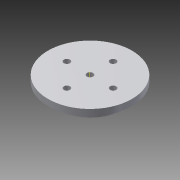
# Autodesk Inventor part: TapaPosterior
Saved by Autodesk Inventor 2013 (Build 170138000, 138)
## iProperties
Created: 2013-06-25
Part Number: TapaPosterior
Material: Genérico
Document SubType Name: Modeling
Designer: usuario
Density: 1 g/cm^3
Author: usuario
Autodesk Inventor part; units mm, degrees
ref_plane "YZ Plane" through (0, 0, 0) normal (1, 0, 0) x (0, 1, 0)
ref_plane "XY Plane" through (0, 0, 0) normal (0, 0, 1) x (1, 0, 0)
sketch "Boceto1" plane through (0, 0, 0) normal (0, 0, 1) x (1, 0, 0)
  circle A0 centre (0, 0) radius 13.5
  dimension "d0" = 27
  constraints: 1 centre point, 1 coincident
  measures "d0" diameter of A0
extrude "Extrusión1" add sketch "Boceto1" along normal blind 2
sketch "Boceto2" plane through (0, 0, 0) normal (0, 0, -1) x (-1, 0, 0)
  circle A0 centre (0, 0) radius 13.5 projected
  circle A1 centre (0, 0) radius 11.23
  dimension "d3" = 22.46
  constraints: 1 centre point, 1 coincident
  measures "d3" diameter of A1
extrude "Extrusión2" add sketch "Boceto2" along normal blind 2 contours A1
sketch "Boceto3" plane through (0, 0, -2) normal (0, 0, -1) x (-1, 0, 0)
  circle A0 centre (0, 0) radius 11.23 projected
  circle A1 centre (0, 0) radius 5.92
  dimension "d6" = 11.84
  constraints: 1 centre point, 1 coincident
  measures "d6" diameter of A1
extrude "Extrusión3" add sketch "Boceto3" along normal blind 2 contours A1
sketch "Boceto4" plane through (0, 0, -4) normal (0, 0, -1) x (-1, 0, 0)
  circle A0 centre (0, 0) radius 5.92 projected
  circle A1 centre (0, 0) radius 3.925
  dimension "d9" = 7.85
  constraints: 1 centre point, 1 coincident
  measures "d9" diameter of A1
extrude "Extrusión4" add sketch "Boceto4" along normal blind 2.5 contours A1
hole "Hole1" at (0, 0, 2) direction (0, 0, -1) diameter 2.02 end through all
hole "Hole2" at (0, 0, -6.5) direction (0, 0, 1) diameter 5.2 depth 2.5
ref_plane "Plano de trabajo1" through (0, 3.925, -4) normal (0, 1, 0) x (-1, 0, 0)
sketch "Boceto11" plane through (0, 3.925, -4) normal (0, 1, 0) x (-1, 0, 0)
  line L0 (0, 9) -> (0, -15.4341)
  line L1 (1.14, 0) -> (-1.14, 0)
  line L2 (-1.14, 0) -> (-1.14, -2.5)
  line L3 (-1.14, -2.5) -> (1.14, -2.5)
  line L4 (1.14, -2.5) -> (1.14, 0)
  dimension "d44" = 2.28
  dimension "d45" = 2.5
  dimension "d46" = 1.14
  constraints: 10 end point, 2 parallel, 2 vertical, 1 horizontal, 1 perpendicular
  measures "d44" distance of L3.end L2.end
  measures "d45" distance of L2.end L1.end
  measures "d46" distance between parallel lines of L0 L2
extrude "Extrusión6" add sketch "Boceto11" along normal blind 1.5 and the other way blind 1
sketch "Boceto13" plane through (0, 0, -2) normal (0, 0, -1) x (-1, 0, 0)
  circle A0 centre (0, 7.4449) radius 1
  constraints: 1 centre point
extrude "Extrusión7" cut sketch "Boceto13" against normal blind 6.5
pattern_circular "Patrón circular2" count 4 over 360 about axis through (0, 0, -10) along (0, 0, 1) of "Extrusión7"
hole "Hole6" at (-7.4449, 0, -4) direction (0, 0, 1) diameter 5.43 depth 2
mirror "Simetría2" about plane through (0, 0, 0) normal (1, 0, 0) of "Hole6"
